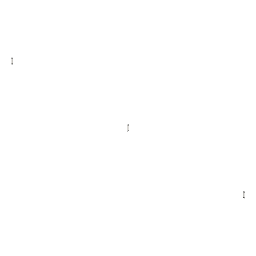
Template Rafix (Autodesk Fusion 360 design; units mm, degrees)
Autodesk Fusion 360 part; units mm, degrees
sketch "ContactArea" plane through (0, 0, 0) normal (0, 0, 1) x (1, 0, 0)
  line L0 (300, -10) -> (-300, -10)
  line L1 (-300, -10) -> (-300, 10)
  line L2 (-300, 10) -> (300, 10)
  line L3 (300, 10) -> (300, -10)
  line L4 (300, -10) -> (-300, 10) construction
  line L5 (-300, -10) -> (300, 10) construction
  dimension "d3" = 600
  dimension "d4" = 20
  constraint horizontal L0
  constraint perpendicular L0 L1
  constraint parallel L0 L2
  constraint parallel L1 L3
  constraint coincident L4 origin
  constraint coincident L5 origin
  measures "d3" distance of L0.start L0.end
  measures "d4" distance of L0 L2
sketch "Sketch2" plane through (0, 0, 0) normal (0, 0, 1) x (1, 0, 0)
  circle A0 centre (240, 0.5) radius 0.5
  line L0 (300, 10) -> (300, -10)
  line L1 (-300, 10) -> (300, 10)
  circle A1 centre (-240, 0.5) radius 0.5
  line L2 (-300, -10) -> (-300, 10)
  dimension "d5" = 1
  dimension "d11" = 60
  dimension "d12" = 9.5
  dimension "d13" = 1
  dimension "d14" = 60
  dimension "d15" = 9.5
  measures "d5" diameter of A0
  measures "d11" distance of A0.centre L0
  measures "d12" distance of A0.centre L1
  measures "d13" diameter of A1
  measures "d14" distance of A1.centre L2
  measures "d15" distance of L1 A1.centre
extrude "Extrude1" add sketch "Sketch2" along normal blind 10 contours A0 makes body 1
pattern_linear "R-Pattern1" count 3 spacing 240 along (-1, 0, 0) of bodies 1 makes body 2 at (0.4994, 0.4751, 6.6667) makes body 3 at (-239.9378, 0.9961, 6.6667)
equation "ContactAreaLength = 600 mm"
equation "ContactAreaWidth = 20 mm"
equation "d3 = ContactAreaLength"
equation "d4 = ContactAreaWidth"
equation "Coord_Y = 9.5 mm"
equation "UserOffset1 = 60 mm"
equation "UserOffset2 = 60 mm"
equation "Offset1 = if(PlacingLength >= MinDistance; UserOffset1; ContactAreaLength / 2)"
equation "Offset2 = if(PlacingLength >= MinDistance; UserOffset2; Offset1)"
equation "d11 = Offset1"
equation "d12 = Coord_Y"
equation "d14 = Offset2"
equation "d15 = Coord_Y"
equation "PlacingLength = ContactAreaLength - UserOffset1 - UserOffset2"
equation "MinDistance = 32 mm"
equation "MaxDistance = 300 mm"
equation "NumberOfIntervals = ceil(PlacingLength / MaxDistance)"
equation "NumberOfComponents = if(PlacingLength >= MinDistance; NumberOfIntervals + 1; 1)"
equation "SpaceBetween = if(PlacingLength >= MinDistance; PlacingLength / NumberOfIntervals; 0 mm)"
equation "d25 = NumberOfComponents"
equation "d27 = SpaceBetween"
